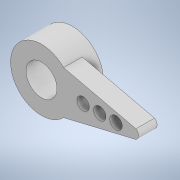
# Autodesk Inventor part: servoarm1
Saved by Autodesk Inventor 2021 (Build 250183000, 183)
## iProperties
Created: 2023-05-31
Part Number: servoarm1
Material: Generic
Document SubType Name: Modeling
Designer: shrus
Density: 1 g/cm^3
Appearance: Default
Author: shrus
Autodesk Inventor part; units mm, degrees
ref_plane "YZ Plane" through (0, 0, 0) normal (1, 0, 0) x (0, 1, 0)
ref_plane "XZ Plane" through (0, 0, 0) normal (0, 1, 0) x (-1, 0, 0)
ref_plane "XY Plane" through (0, 0, 0) normal (0, 0, 1) x (1, 0, 0)
sketch "Sketch1" plane through (0, 0, 0) normal (0, 0, 1) x (1, 0, 0)
  circle A0 centre (-5.565, 4.9924) radius 5
  circle A1 centre (-5.565, 4.9924) radius 2.5
  point P0 (0, 0)
  dimension "d0" = 10
  dimension "d1" = 5
  constraints: 2 centre point, 1 coincident
  measures "d0" diameter of A0
  measures "d1" diameter of A1
extrude "Extrusion1" add sketch "Sketch1" along normal blind 5
sketch "Sketch2" plane through (-5.565, 4.9924, 5) normal (0, 0, 1) x (1, 0, 0)
  line L0 (3.5707, 3.5) -> (3.5707, -3.5)
  circle A0 centre (0, 0) radius 5 projected
  line L1 (3.5707, 3.5) -> (15.2599, 0.7864)
  line L2 (15.2599, -0.7136) -> (3.5707, -3.5)
  arc A1 (15.2599, -0.7136) -> (15.2599, 0.7864) centre (14.7767, 0.0364) ccw
  circle A2 centre (6.7246, 0.0364) radius 1
  circle A3 centre (9.4153, 0.0364) radius 1
  circle A4 centre (12.048, 0.0364) radius 1
  point P0 (5.565, -4.9924)
  point P1 (5, 0)
  dimension "d8" = 2
  dimension "d9" = 2
  dimension "d10" = 2
  constraints: 6 end point, 4 centre point, 3 point on circle, 1 point on line
  measures "d8" diameter of A2
  measures "d9" diameter of A3
  measures "d10" diameter of A4
extrude "Extrusion2" add sketch "Sketch2" against normal blind 3 contours L1 A1 L2 A0
body "Solid1"
